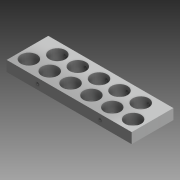
# Autodesk Inventor part: Ventilhalter
Saved by Autodesk Inventor 2013 (Build 170138000, 138)
## iProperties
Created: 2012-07-24
Part Number: Ventilhalter
Material: Aluminium 6061
Document SubType Name: Modeling
Designer: fivef
Density: 1 g/cm^3
Author: fivef
Autodesk Inventor part; units mm, degrees
ref_plane "YZ Plane" through (0, 0, 0) normal (1, 0, 0) x (0, 1, 0)
ref_plane "XZ Plane" through (0, 0, 0) normal (0, 1, 0) x (-1, 0, 0)
ref_plane "XY Plane" through (0, 0, 0) normal (0, 0, 1) x (1, 0, 0)
sketch "Skizze1" plane through (0, 0, 0) normal (0, 0, 1) x (1, 0, 0)
  circle A0 centre (0, 0) radius 11.5
  circle A1 centre (15, 25.9808) radius 11.5
  circle A2 centre (30, 0) radius 11.5
  circle A3 centre (44.4291, 25.9808) radius 11.5
  circle A4 centre (60, 0) radius 11.5
  circle A5 centre (75, 25.9615) radius 11.5
  circle A6 centre (90, -0.0192) radius 11.5
  circle A7 centre (104.4291, 25.9615) radius 11.5
  circle A8 centre (120, 0) radius 11.5
  circle A9 centre (135, 25.9615) radius 11.5
  circle A10 centre (150, -0.0192) radius 11.5
  line L0 (-15, 42.9808) -> (165, 42.9808)
  line L1 (165, 42.9808) -> (165, -17.0192)
  line L2 (165, -17.0192) -> (-15, -17.0192)
  line L3 (-15, -17.0192) -> (-15, 42.9808)
  dimension "d0" = 23
  dimension "d2" = 23
  dimension "d3" = 30
  dimension "d4" = 23
  dimension "d7" = 30
  dimension "d8" = 30
  dimension "d9" = 23
  dimension "d10" = 29.4291
  dimension "d11" = 23
  dimension "d12" = 23
  dimension "d13" = 23
  dimension "d14" = 30
  dimension "d15" = 23
  dimension "d16" = 29.4291
  dimension "d24" = 23
  dimension "d25" = 23
  dimension "d26" = 23
  dimension "d27" = 30
  dimension "d28" = 15
  dimension "d31" = 15
  dimension "d36" = 180
  dimension "d98" = 60
  dimension "d99" = 5.5
  dimension "d100" = 52.4567
  dimension "d101" = 5.5192
  dimension "d102" = 5.5
  dimension "d103" = 5.5
  constraints: 11 centre point, 8 end point, 2 parallel, 1 coincident, 1 horizontal, 1 horizontal alignment, 1 perpendicular
  measures "d0" diameter of A0
  measures "d2" diameter of A1
  measures "d3" distance of A1.centre point (0, 0)
  measures "d4" diameter of A2
  measures "d7" distance of A2.centre A1.centre
  measures "d8" distance of A2.centre point (0, 0)
  measures "d9" diameter of A3
  measures "d10" distance of A3.centre A1.centre
  measures "d11" diameter of A4
  measures "d12" diameter of A5
  measures "d13" diameter of A6
  measures "d14" distance of A6.centre A5.centre
  measures "d15" diameter of A7
  measures "d16" distance of A7.centre A5.centre
  measures "d24" diameter of A8
  measures "d25" diameter of A9
  measures "d26" diameter of A10
  measures "d27" distance of A10.centre A9.centre
  measures "d28" distance from line of L3 A0.centre
  measures "d31" distance from line of L1 A10.centre
  measures "d36" distance of L0.end L0.start
  measures "d98" distance between parallel lines of L0 L2
  measures "d99" distance edge to line of A1 L0
  measures "d100" distance of A7.centre A10.centre
  measures "d101" distance edge to line of A4 L2
  measures "d102" distance edge to line of A6 L2
  measures "d103" distance edge to line of A10 L2
extrude "Extrusion1" add sketch "Skizze1" along normal blind 15
hole "Bohrung1" at (120, -17.0192, 7.5) at (30, -17.0192, 7.5) at (0, -17.0192, 7.5) at (60, -17.0192, 7.5) at (150, -17.0192, 7.5) at (90, -17.0192, 7.5) direction (0, 1, 0) diameter 4 depth 8
thread "Gewinde2" size "M4x0.7" class "6H" standard "ANSI Metric M Profile" full length
thread "Gewinde3" size "M4x0.7" class "6H" standard "ANSI Metric M Profile" full length
sketch "Skizze4" plane through (-15, 42.9808, 0) normal (0, 1, 0) x (1, 0, 0)
  line L0 (180, 0) -> (180, -15) projected
  line L1 (150, 13) -> (150, -28.8024) construction
  line L2 (30, 13) -> (30, -28.8024) construction
  line L3 (119.4291, 13) -> (119.4291, -28.8024) construction
  line L4 (90, 13) -> (90, -28.8024) construction
  line L5 (59.4291, 13) -> (59.4291, -28.8024) construction
  line L6 (180, -15) -> (0, -15) projected
  line L7 (0, -15) -> (180, 0) construction
  line L8 (180, -15) -> (0, 0) construction
  line L9 (4.4998, -7.5) -> (175.5002, -7.5) construction
  point P0 (15, 0)
  point P1 (119.4291, -7.5)
  point P2 (150, -7.5)
  point P3 (90, -7.5)
  point P4 (59.4291, -7.5)
  point P5 (30, -7.5)
  point P6 (90, -7.5)
  point P7 (90, -7.5)
  dimension "d58" = 30
  dimension "d60" = 60.5709
  dimension "d62" = 90
  dimension "d64" = 120.5709
  dimension "d66" = 150
  dimension "d85" = 0
  dimension "d86" = 0
  dimension "d87" = 0
  dimension "d88" = 0
  dimension "d89" = 0
  constraints: 6 end point, 2 midpoint, 1 parallel
  measures "d58" distance from line of point (150, -7.5) L0
  measures "d60" distance from line of point (119.429, -7.5) L0
  measures "d62" distance from line of point (90, -7.5) L0
  measures "d64" distance from line of point (59.429, -7.5) L0
  measures "d66" distance from line of point (30, -7.5) L0
  measures "d85" distance from line of L9 point (30, -7.5)
  measures "d86" distance from line of L9 point (59.429, -7.5)
  measures "d87" distance from line of L9 point (90, -7.5)
  measures "d88" distance from line of L9 point (119.429, -7.5)
  measures "d89" distance from line of L9 point (150, -7.5)
hole "Bohrung2" at (104.4291, 42.9808, 7.5) at (135, 42.9808, 7.5) at (75, 42.9808, 7.5) at (44.4291, 42.9808, 7.5) at (15, 42.9808, 7.5) direction (0, -1, 0) diameter 4 depth 8 tip angle 118
thread "Gewinde4" size "M4x0.7" class "6H" standard "ANSI Metric M Profile" full length
thread "Gewinde5" size "M4x0.7" class "6H" standard "ANSI Metric M Profile" full length
thread "Gewinde6" size "M4x0.7" class "6H" standard "ANSI Metric M Profile" full length
thread "Gewinde7" size "M4x0.7" class "6H" standard "ANSI Metric M Profile" full length
thread "Gewinde8" size "M4x0.7" class "6H" standard "ANSI Metric M Profile" full length
